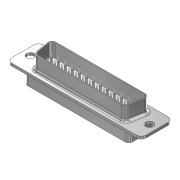
# Autodesk Inventor part: D-SUB Male
Saved by Autodesk Inventor 2015 (Build 190159000, 159)
## iProperties
Created: 2012-07-04
Part Number: D-SUB Male
Material: Steel
Document SubType Name: Modeling
Density: 7.85 g/cm^3
Mass: 22.2866 g
Surface Area: 31.3439 cm^2
Volume: 2.83906 cm^3
Appearance: Chrome - Polished
Categories: <MemberInstance><Categories><Category DisplayName="" Mnemonic="CABLEANDHARNESS" InternalName="e4a7e005-5e42-4d16-b293-125e7f0d0512"><Category DisplayName="" Mnemonic="CONNECTORS" InternalName="6f634eba-a678-4820-a31d-2c2d5ee6728e"><CategoryParameter DisplayName="" Mnemonic="REFDES" InternalName="c3740e8c-60ab-4d5d-8584-52b73222f2f0"/><Category DisplayName="" Mnemonic="DISCRETEWIRE" InternalName="9a3407de-09b2-4cdb-8c40-9708d5144a28"/></Category></Category></Categories><FamilyTemplate><FamilyTemplateParameters></FamilyTemplateParameters></FamilyTemplate><CategoryParameterMap><ParamToTemplateMap><ParamToTemplate CategoryParameter="//CategoryParameter[@InternalName='c3740e8c-60ab-4d5d-8584-52b73222f2f0']" ConstantValue=""/></ParamToTemplateMap></CategoryParameterMap></MemberInstance>
Autodesk Inventor part; units mm, degrees
ref_plane "YZ Plane" through (0, 0, 0) normal (1, 0, 0) x (0, 1, 0)
ref_plane "XZ Plane" through (0, 0, 0) normal (0, 1, 0) x (-1, 0, 0)
ref_plane "XY Plane" through (0, 0, 0) normal (0, 0, 1) x (1, 0, 0)
sketch "Sketch1" plane through (0, 0, 0) normal (0, 0, 1) x (1, 0, 0)
  line L0 (-24.52, 6.275) -> (24.52, 6.275)
  line L1 (26.52, 4.275) -> (26.52, -4.275)
  line L2 (24.52, -6.275) -> (-24.52, -6.275)
  line L3 (-26.52, -4.275) -> (-26.52, 4.275)
  line L4 (-19.1696, 2.4195) -> (-18.2245, -2.9405)
  line L5 (-16.7473, -4.18) -> (16.7473, -4.18)
  line L6 (18.2245, -2.9405) -> (19.1696, 2.4195)
  line L7 (17.6924, 4.18) -> (-17.6924, 4.18)
  line L8 (-23.52, 0) -> (23.52, 0) construction
  line L9 (-1.385, -1.42) -> (1.385, -1.42) construction
  line L10 (0, 1.42) -> (0, -1.42) construction
  arc A0 (-24.52, 6.275) -> (-26.52, 4.275) centre (-24.52, 4.275) ccw
  arc A1 (-26.52, -4.275) -> (-24.52, -6.275) centre (-24.52, -4.275) ccw
  arc A2 (24.52, -6.275) -> (26.52, -4.275) centre (24.52, -4.275) ccw
  arc A3 (26.52, 4.275) -> (24.52, 6.275) centre (24.52, 4.275) ccw
  arc A4 (-17.6924, 4.18) -> (-19.1696, 2.4195) centre (-17.6924, 2.68) ccw
  arc A5 (-18.2245, -2.9405) -> (-16.7473, -4.18) centre (-16.7473, -2.68) ccw
  arc A6 (16.7473, -4.18) -> (18.2245, -2.9405) centre (16.7473, -2.68) ccw
  arc A7 (19.1696, 2.4195) -> (17.6924, 4.18) centre (17.6924, 2.68) ccw
  line L11 (0, 4.18) -> (0, -4.18) construction
  circle A8 centre (0, 1.42) radius 0.5
  circle A9 centre (1.385, -1.42) radius 0.5
  circle A10 centre (-1.385, -1.42) radius 0.5
  line L12 (-19.15, 5.36) -> (19.15, 5.36)
  line L13 (20.65, 3.86) -> (20.65, -3.86)
  line L14 (19.15, -5.36) -> (-19.15, -5.36)
  line L15 (-20.65, -3.86) -> (-20.65, 3.86)
  arc A11 (-19.15, 5.36) -> (-20.65, 3.86) centre (-19.15, 3.86) ccw
  arc A12 (-20.65, -3.86) -> (-19.15, -5.36) centre (-19.15, -3.86) ccw
  arc A13 (19.15, -5.36) -> (20.65, -3.86) centre (19.15, -3.86) ccw
  arc A14 (20.65, 3.86) -> (19.15, 5.36) centre (19.15, 3.86) ccw
  point P0 (0, 0)
  point P1 (-26.52, 6.275)
  point P2 (26.52, 6.275)
  point P3 (-26.52, -6.275)
  point P4 (0, 6.275)
  point P5 (26.52, 0)
  point P6 (-19.48, 4.18)
  point P7 (19.48, 4.18)
  point P8 (18.697, -0.2605)
  point P9 (0, 0)
  point P10 (0, 0)
  point P11 (0, 0)
  point P12 (-20.65, 5.36)
  point P13 (20.65, -5.36)
  point P14 (20.65, 5.36)
  point P15 (0, 5.36)
  point P16 (20.65, 0)
  dimension "d0" = 53.04
  dimension "d1" = 12.55
  dimension "d2" = 8.36
  dimension "d3" = 38.96
  dimension "d4" = 80
  dimension "d5" = 47.04
  dimension "d6" = 2.77
  dimension "d7" = 2.84
  dimension "d8" = 2
  dimension "d9" = 1.5
  dimension "d25" = 1
  dimension "d42" = 41.3
  dimension "d43" = 10.72
  dimension "d44" = 1.5
  constraints: 32 end point, 24 point on circle, 24 tangent, 16 point on line, 15 centre point, 11 equal radius, 11 midpoint, 7 parallel, 6 coincident, 6 vertical alignment, 5 perpendicular, 4 horizontal alignment, 2 horizontal
  measures "d0" distance of point (-26.52, 6.275) point (26.52, 6.275)
  measures "d1" distance of point (-26.52, -6.275) point (-26.52, 6.275)
  measures "d2" distance between parallel lines of L5 L7
  measures "d3" distance of point (19.48, 4.18) point (-19.48, 4.18)
  measures "d4" angle of L7 L4
  measures "d5" distance of L8.start L8.end
  measures "d6" distance of L9.end L9.start
  measures "d7" distance from line of L10.start L9
  measures "d8" radius of A0
  measures "d9" radius of A4
  measures "d25" diameter of A8
  measures "d42" distance of point (-20.65, 5.36) point (20.65, 5.36)
  measures "d43" distance of point (20.65, 5.36) point (20.65, -5.36)
  measures "d44" radius of A11
extrude "Extrusion1" add sketch "Sketch1" along normal blind 1 contours L0 A3 L1 A2 L2 A1 L3 A0 | A4 L7 A7 L6 A6 L5 A5 L4 | A8 | A9 | A10 | L12 A14 L13 A13 L14 A12 L15 A11
extrude "Extrusion2" add sketch "Sketch1" along normal blind 6.5 contours A4 L7 A7 L6 A6 L5 A5 L4 | A8 | A9 | A10
sketch "Sketch2" plane through (0, 0, 6.5) normal (0, 0, 1) x (1, 0, 0)
  arc A0 (-17.6924, 4.18) -> (-19.1696, 2.4195) centre (-17.6924, 2.68) ccw projected
  line L0 (-18.2245, -2.9405) -> (-19.1696, 2.4195) projected
  arc A1 (-18.2245, -2.9405) -> (-16.7473, -4.18) centre (-16.7473, -2.68) ccw projected
  line L1 (16.7473, -4.18) -> (-16.7473, -4.18) projected
  arc A2 (16.7473, -4.18) -> (18.2245, -2.9405) centre (16.7473, -2.68) ccw projected
  line L2 (19.1696, 2.4195) -> (18.2245, -2.9405) projected
  arc A3 (19.1696, 2.4195) -> (17.6924, 4.18) centre (17.6924, 2.68) ccw projected
  line L3 (-17.6924, 4.18) -> (17.6924, 4.18) projected
  arc A4 (18.8741, 2.4716) -> (17.6924, 3.88) centre (17.6924, 2.68) ccw
  line L4 (18.8741, 2.4716) -> (17.929, -2.8884)
  arc A5 (16.7473, -3.88) -> (17.929, -2.8884) centre (16.7473, -2.68) ccw
  line L5 (16.7473, -3.88) -> (-16.7473, -3.88)
  arc A6 (-17.929, -2.8884) -> (-16.7473, -3.88) centre (-16.7473, -2.68) ccw
  line L6 (-17.929, -2.8884) -> (-18.8741, 2.4716)
  arc A7 (-17.6924, 3.88) -> (-18.8741, 2.4716) centre (-17.6924, 2.68) ccw
  line L7 (-17.6924, 3.88) -> (17.6924, 3.88)
  point P0 (0, 0)
  dimension "d22" = 0.3
  constraints: 8 end point, 8 point on circle, 4 centre point, 7 other
  measures "d22" distance between parallel lines of L3 L7
extrude "Extrusion3" cut sketch "Sketch2" against normal up to surface (5.5 mm away) contours L4 A5 L5 A6 L6 A7 L7 A4
extrude "Extrusion4" add sketch "Sketch1" along normal blind 5.5 contours A8
extrude "Extrusion5" add sketch "Sketch1" along normal blind 5.5 contours A9 | A10
chamfer "Chamfer1" distance 0.4 angle 80 1 edges at (-0.5, 1.42, 5.5) measured on face at (-0.0947, 1.2828, 5.5)
chamfer "Chamfer2" distance 0.4 angle 80 1 edges at (0.885, -1.42, 5.5) measured on face at (1.2903, -1.5572, 5.5)
chamfer "Chamfer3" distance 0.4 angle 80 1 edges at (-1.885, -1.42, 5.5) measured on face at (-1.4797, -1.5572, 5.5)
pattern_linear "Rectangular Pattern1" count 13 spacing 2.77 along (1, 0, 0) of "Extrusion4", "Chamfer1" first direction both ways yes
hole "Hole1" at (-23.52, 0, 0) at (23.52, 0, 0) direction (0, 0, 1) diameter 3.05 end through all
extrude "Extrusion6" add sketch "Sketch1" against normal blind 4.5 contours A4 L7 A7 L6 A6 L5 A5 L4 | A8 | A9 | A10 | L12 A14 L13 A13 L14 A12 L15 A11
pattern_linear "Rectangular Pattern2" count 6 spacing 2.77 along (1, 0, 0) of "Extrusion5", "Chamfer3", "Chamfer2"
pattern_linear "Rectangular Pattern3" count 6 spacing 2.77 along (-1, 0, 0) of "Extrusion5", "Chamfer3", "Chamfer2"
fillet "Fillet1" radius 1 8 edges at (-17.7114, -3.8291, 1) (-18.697, -0.2605, 1) (-18.8414, 3.6442, 1) (0, 4.18, 1) (18.8414, 3.6442, 1) (18.697, -0.2605, 1) (17.7114, -3.8291, 1) (0, -4.18, 1)
sketch "Sketch3" plane through (0, 0, -4.5) normal (0, 0, -1) x (-1, 0, 0)
  circle A0 centre (-16.62, 1.42) radius 0.1 projected
  circle A1 centre (-15.235, -1.42) radius 0.1 projected
  point P0 (0, 0)
  constraints: 2 coincident
equation "\"d41\" = d6"
equation "\"d49\" = d6"
equation "\"d52\" = d6"
body "Solid1"
